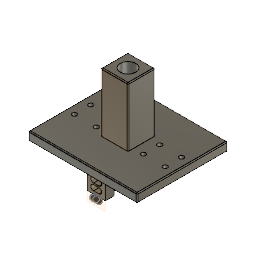
camera_house (Autodesk Fusion 360 design; units mm, degrees)
Autodesk Fusion 360 part; units mm, degrees
sketch "Sketch1" plane through (0, 0, 0) normal (0, 0, 1) x (1, 0, 0)
  line L0 (0, 0) -> (120, 0)
  line L1 (120, 0) -> (120, 100)
  line L2 (120, 100) -> (0, 100)
  line L3 (0, 100) -> (0, 0)
  line L4 (60, 100) -> (60, 0)
  line L5 (98, 100) -> (98, 0)
  line L6 (22, 100) -> (22, 0)
  line L7 (22, 50) -> (10, 50)
  line L8 (10, 50) -> (10, 59)
  line L9 (10, 59) -> (22, 59)
  line L10 (22, 59) -> (22, 50)
  circle A0 centre (10, 59) radius 2.5
  line L11 (22, 50) -> (34, 50)
  line L12 (34, 50) -> (34, 59)
  line L13 (34, 59) -> (22, 59)
  line L14 (22, 59) -> (22, 50)
  line L15 (10, 50) -> (34, 50)
  line L16 (34, 50) -> (34, 41)
  line L17 (34, 41) -> (10, 41)
  line L18 (10, 41) -> (10, 50)
  circle A1 centre (10, 41) radius 2.5
  circle A2 centre (34, 41) radius 2.5
  circle A3 centre (34, 59) radius 2.5
  line L19 (60, 50) -> (120, 50)
  line L20 (98, 50) -> (110, 50)
  line L21 (110, 50) -> (110, 59)
  line L22 (110, 59) -> (98, 59)
  line L23 (98, 59) -> (98, 50)
  line L24 (98, 50) -> (86, 50)
  line L25 (86, 50) -> (86, 59)
  line L26 (86, 59) -> (98, 59)
  line L27 (98, 59) -> (98, 50)
  line L28 (86, 50) -> (110, 50)
  line L29 (110, 50) -> (110, 41)
  line L30 (110, 41) -> (86, 41)
  line L31 (86, 41) -> (86, 50)
  circle A4 centre (86, 59) radius 2.5
  circle A5 centre (110, 59) radius 2.5
  circle A6 centre (86, 41) radius 2.5
  circle A7 centre (110, 41) radius 2.5
  dimension "d1" = 120
  dimension "d2" = 100
  dimension "d3" = 38
  dimension "d4" = 38
  dimension "d6" = 5
  dimension "d7" = 24
  dimension "d8" = 18
  dimension "d9" = 5
  dimension "d10" = 5
  dimension "d11" = 5
  dimension "d12" = 9
  dimension "d13" = 12
  dimension "d14" = 9
  dimension "d15" = 12
  dimension "d16" = 24
  dimension "d17" = 9
  dimension "d18" = 5
  dimension "d19" = 5
  dimension "d20" = 5
  dimension "d21" = 5
  constraint horizontal L0
  constraint vertical L1
  constraint horizontal L2
  constraint vertical L3
  constraint coincident L0.start L3.end
  constraint midpoint L2 L4.start
  constraint midpoint L0 L4.end
  constraint coincident L2 L5.start
  constraint coincident L0 L5.end
  constraint perpendicular L0 L5
  constraint coincident L2 L6.start
  constraint coincident L0 L6.end
  constraint perpendicular L0 L6
  constraint horizontal L7
  constraint vertical L8
  constraint horizontal L9
  constraint vertical L10
  constraint midpoint L6 L7.start
  constraint coincident L8.end L9.start
  constraint horizontal L11
  constraint vertical L12
  constraint horizontal L13
  constraint vertical L14
  constraint horizontal L15
  constraint vertical L16
  constraint horizontal L17
  constraint vertical L18
  constraint coincident L17.end L18.start
  constraint coincident L16.end L17.start
  constraint coincident L12.end L13.start
  constraint midpoint L4 L19.start
  constraint midpoint L1 L19.end
  constraint horizontal L20
  constraint vertical L21
  constraint horizontal L22
  constraint vertical L23
  constraint midpoint L5 L20.start
  constraint horizontal L24
  constraint vertical L25
  constraint horizontal L26
  constraint vertical L27
  constraint horizontal L28
  constraint vertical L29
  constraint horizontal L30
  constraint vertical L31
  constraint coincident L25.end L26.start
  constraint coincident L21.end L22.start
  constraint coincident L30.end L31.start
  constraint coincident L29.end L30.start
  measures "d1" distance of L0.start L0.end
  measures "d2" distance of L0.start L2.end
  measures "d3" distance of L4 L5
  measures "d4" distance of L4 L6
  measures "d6" diameter of A0
  measures "d7" distance of L8 L12
  measures "d8" distance of L9 L17
  measures "d9" diameter of A1
  measures "d10" diameter of A2
  measures "d11" diameter of A3
  measures "d12" distance of L20.start L22.end
  measures "d13" distance of L20.start L20.end
  measures "d14" distance of L20.start L22.end
  measures "d15" distance of L20.start L24.end
  measures "d16" distance of L24.end L20.end
  measures "d17" distance of L24.end L30.end
  measures "d18" diameter of A4
  measures "d19" diameter of A5
  measures "d20" diameter of A6
  measures "d21" diameter of A7
  measures "d40" diameter of L0.end
extrude "Extrude1" add sketch "Sketch1" along normal blind 10 contours L0 L2 L3 L6 L8 L9 A0 L17 L18 A1 | L0 L2 L4 L6 L12 L13 L16 L17 A2 A3 | L0 L4 L5 L19 L30 L31 A6 | L6 L7 L15 L17 L18 A1 | L6 L11 L15 L16 L17 A2 | L0 L1 L5 L19 L29 L30 A7 | L2 L4 L5 L19 L25 L26 A4 | L6 L7 L8 L9 L10 A0 L14 L15 | L6 L10 L11 L12 L13 L14 L15 A3 | L5 L19 L24 L28 L30 L31 A6 | L5 L19 L20 L28 L29 L30 A7 | L5 L19 L23 L24 L25 L26 L27 L28 A4 | L1 L2 L5 L19 L21 L22 A5 | L5 L19 L20 L21 L22 L23 L27 L28 A5
sketch "Sketch2" plane through (0, 0, 0) normal (0, 0, -1) x (1, 0, 0)
  circle A0 centre (110, -41) radius 2.5
  circle A1 centre (86, -59) radius 2.5
  circle A2 centre (10, -59) radius 2.5
  circle A3 centre (110, -59) radius 2.5
  circle A4 centre (86, -41) radius 2.5
  circle A5 centre (10, -41) radius 2.5
  circle A6 centre (34, -41) radius 2.5
  circle A7 centre (34, -59) radius 2.5
  line L0 (0, 0) -> (0, -100)
  line L1 (0, -100) -> (120, -100)
  line L2 (120, -100) -> (120, 0)
  line L3 (120, 0) -> (0, 0)
  line L4 (0, -50) -> (120, -50)
  line L5 (60, -100) -> (60, 0)
  line L6 (0, -85) -> (120, -85)
  line L7 (60, -85) -> (70, -85)
  line L8 (70, -85) -> (70, -75)
  line L9 (70, -75) -> (60, -75)
  line L10 (60, -75) -> (60, -85)
  line L11 (60, -85) -> (50, -85)
  line L12 (50, -85) -> (50, -75)
  line L13 (50, -75) -> (60, -75)
  line L14 (60, -75) -> (60, -85)
  line L15 (0, -15) -> (120, -15)
  line L16 (60, -15) -> (70, -15)
  line L17 (70, -15) -> (70, -25)
  line L18 (70, -25) -> (60, -25)
  line L19 (60, -25) -> (60, -15)
  line L20 (60, -25) -> (50, -25)
  line L21 (50, -25) -> (50, -15)
  line L22 (50, -15) -> (60, -15)
  line L23 (60, -15) -> (60, -25)
  dimension "d24" = 15
  dimension "d25" = 10
  dimension "d26" = 10
  dimension "d27" = 10
  dimension "d28" = 15
  dimension "d29" = 10
  dimension "d30" = 10
  dimension "d31" = 10
  dimension "d32" = 10
  constraint midpoint L0 L4.start
  constraint midpoint L2 L4.end
  constraint midpoint L1 L5.start
  constraint midpoint L3 L5.end
  constraint coincident L0 L6.start
  constraint coincident L2 L6.end
  constraint horizontal L7
  constraint vertical L8
  constraint horizontal L9
  constraint vertical L10
  constraint midpoint L6 L7.start
  constraint horizontal L11
  constraint vertical L12
  constraint horizontal L13
  constraint vertical L14
  constraint coincident L0 L15.start
  constraint coincident L2 L15.end
  constraint horizontal L16
  constraint vertical L17
  constraint horizontal L18
  constraint vertical L19
  constraint midpoint L15 L16.start
  constraint horizontal L20
  constraint vertical L21
  constraint horizontal L22
  constraint vertical L23
  measures "d24" distance of L1 L6
  measures "d25" distance of L7.start L7.end
  measures "d26" distance of L7.start L9.end
  measures "d27" distance of L7.start L9.end
  measures "d28" distance of L3 L15
  measures "d29" distance of L16.start L16.end
  measures "d30" distance of L16.start L18.end
  measures "d31" distance of L18.end L20.end
  measures "d32" distance of L18.end L16.start
extrude "Extrude2" add sketch "Sketch2" along normal blind 20 contours L5 L15 L19 L20 L21 L22 L23 | L5 L15 L16 L17 L18 L19 L23 | L5 L6 L10 L11 L12 L13 L14 | L5 L6 L7 L8 L9 L10 L14
extrude "Extrude3" add 2 faces at (56.6667, 18.3333, -20) (56.6667, 78.3333, -20) along direction (0, 0, -1) blind 10
sketch "Sketch6" plane through (0, 15, 0) normal (0, -1, 0) x (1, 0, 0)
  line L0 (70, 0) -> (50, 0)
  line L1 (50, 0) -> (50, -30)
  line L2 (50, -30) -> (70, -30)
  line L3 (70, -30) -> (70, 0)
  line L4 (50, -15.9999) -> (70, -16)
  line L5 (56.995, -26.5146) -> (62.9949, -26.5247)
  arc A0 (62.9949, -26.5247) -> (63.0051, -20.5247) centre (63, -23.5247) ccw
  line L6 (63.0051, -20.5247) -> (57.0051, -20.5146)
  arc A1 (57.0051, -20.5146) -> (56.995, -26.5146) centre (57, -23.5146) ccw
  line L7 (50, -23.5028) -> (54, -23.5096)
  line L8 (66, -23.5298) -> (70, -23.5365)
  line L9 (57, -11.4803) -> (63, -11.4803)
  arc A2 (63, -11.4803) -> (63, -5.4803) centre (63, -8.4803) ccw
  line L10 (63, -5.4803) -> (57, -5.4803)
  arc A3 (57, -5.4803) -> (57, -11.4803) centre (57, -8.4803) ccw
  line L11 (50, -8.4803) -> (54, -8.4803)
  line L12 (66, -8.4803) -> (70, -8.4803)
  point P0 (60, -23.5197)
  point P1 (60, -8.4803)
  dimension "d40" = 6
  dimension "d41" = 6
  constraint coincident L1 L4.start
  constraint coincident L3 L4.end
  constraint coincident L1 L11.start
  constraint coincident L3 L12.end
  constraint perpendicular L3 L11
  constraint coincident L1 L7.start
  constraint coincident L3 L8.end
  constraint tangent L5 A0
  constraint tangent A0 L6
  constraint parallel L5 L6
  constraint tangent L6 A1
  constraint tangent L5 A1
  constraint coincident A1 L7.end
  constraint coincident A0 L8.start
  constraint collinear L7 L8
  constraint coincident P0 L7
  constraint tangent L9 A2
  constraint tangent A2 L10
  constraint parallel L9 L10
  constraint tangent L10 A3
  constraint tangent L9 A3
  constraint coincident A3 L11.end
  constraint coincident A2 L12.start
  constraint collinear L11 L12
  constraint coincident P1 L11
  measures "d40" diameter of A0
  measures "d41" diameter of A2
extrude "Extrude4" cut sketch "Sketch6" against normal blind 200 contours L9 A2 L10 A3 | L5 A0 L6 A1
extrude "Extrude5" add 2 faces at (56.6667, 78.3333, -30) (56.6667, 18.3333, -30) along direction (0, 0, -1) blind 10
sketch "Sketch7" plane through (0, 15, 0) normal (0, -1, 0) x (1, 0, 0)
  line L0 (63, -11.4803) -> (57, -11.4803)
  arc A0 (57, -5.4803) -> (57, -11.4803) centre (57, -8.4803) ccw
  line L1 (57, -5.4803) -> (63, -5.4803)
  arc A1 (63, -11.4803) -> (63, -5.4803) centre (63, -8.4803) ccw
  line L2 (62.9949, -26.5247) -> (56.995, -26.5146)
  arc A2 (57.0051, -20.5146) -> (56.995, -26.5146) centre (57, -23.5146) ccw
  line L3 (57.0051, -20.5146) -> (63.0051, -20.5247)
  arc A3 (62.9949, -26.5247) -> (63.0051, -20.5247) centre (63, -23.5247) ccw
  line L4 (70, 0) -> (50, 0)
  line L5 (50, 0) -> (50, -40)
  line L6 (50, -40) -> (70, -40)
  line L7 (70, -40) -> (70, 0)
  line L8 (57, -36) -> (63, -36)
  arc A4 (63, -36) -> (63, -30) centre (63, -33) ccw
  line L9 (63, -30) -> (57, -30)
  arc A5 (57, -30) -> (57, -36) centre (57, -33) ccw
  line L10 (57, -33) -> (63, -33) construction
  point P0 (60, -33)
  dimension "d46" = 6
  constraint tangent L8 A4
  constraint tangent A4 L9
  constraint parallel L8 L9
  constraint tangent L9 A5
  constraint tangent L8 A5
  constraint horizontal L10
  constraint midpoint L10 P0
  measures "d46" diameter of A4
sketch "Sketch8" plane through (0, 0, 10) normal (0, 0, 1) x (-1, 0, 0)
  circle A0 centre (-110, -41) radius 2.5
  circle A1 centre (-86, -59) radius 2.5
  circle A2 centre (-10, -59) radius 2.5
  circle A3 centre (-110, -59) radius 2.5
  circle A4 centre (-86, -41) radius 2.5
  circle A5 centre (-10, -41) radius 2.5
  circle A6 centre (-34, -41) radius 2.5
  circle A7 centre (-34, -59) radius 2.5
  line L0 (0, -100) -> (0, 0)
  line L1 (0, 0) -> (-120, 0)
  line L2 (-120, 0) -> (-120, -100)
  line L3 (-120, -100) -> (0, -100)
  line L4 (-60, 0) -> (-60, -100)
  line L5 (0, -50) -> (-120, -50)
  line L6 (-86, -59) -> (-86, -100)
  line L7 (-80.75, -100) -> (-80.75, -11.2422)
  line L8 (-60, -50) -> (-75, -50)
  line L9 (-75, -50) -> (-75, -65)
  line L10 (-75, -65) -> (-60, -65)
  line L11 (-60, -65) -> (-60, -50)
  line L12 (-60, -50) -> (-45, -50)
  line L13 (-45, -50) -> (-45, -65)
  line L14 (-45, -65) -> (-60, -65)
  line L15 (-60, -65) -> (-60, -50)
  line L16 (-45, -50) -> (-75, -50)
  line L17 (-75, -50) -> (-75, -35)
  line L18 (-75, -35) -> (-45, -35)
  line L19 (-45, -35) -> (-45, -50)
  dimension "d51" = 26
  dimension "d52" = 5.25
  dimension "d53" = 30
  dimension "d54" = 15
  constraint midpoint L1 L4.start
  constraint midpoint L3 L4.end
  constraint midpoint L0 L5.start
  constraint midpoint L2 L5.end
  constraint coincident A1.centre L6.start
  constraint coincident L3 L6.end
  constraint perpendicular L3 L6
  constraint coincident L3 L7.start
  constraint perpendicular L3 L7
  constraint horizontal L8
  constraint vertical L9
  constraint horizontal L10
  constraint vertical L11
  constraint midpoint L4 L8.start
  constraint horizontal L12
  constraint vertical L13
  constraint horizontal L14
  constraint vertical L15
  constraint horizontal L16
  constraint vertical L17
  constraint horizontal L18
  constraint vertical L19
  measures "d51" distance of A4.centre L4
  measures "d52" distance of L6 L7
  measures "d53" distance of L12.end L8.end
  measures "d54" distance of L12.end L18.end
extrude "Extrude8" add sketch "Sketch8" along normal blind 65 contours L4 L5 L11 L12 L13 L14 L15 L16 | L4 L5 L12 L16 L18 L19 | L4 L5 L8 L9 L10 L11 L15 L16 | L4 L5 L8 L16 L17 L18
sketch "Sketch9" plane through (0, 0, 75) normal (0, 0, 1) x (-1, 0, 0)
  line L0 (-75, -35) -> (-75, -65)
  line L1 (-75, -65) -> (-45, -65)
  line L2 (-45, -65) -> (-45, -35)
  line L3 (-45, -35) -> (-75, -35)
  line L4 (-60, -35) -> (-60, -65)
  line L5 (-45, -50) -> (-75, -50)
  circle A0 centre (-60, -50) radius 8.5
  dimension "d57" = 17
  constraint midpoint L3 L4.start
  constraint midpoint L1 L4.end
  constraint midpoint L2 L5.start
  constraint midpoint L0 L5.end
  constraint midpoint L5 A0.centre
  measures "d57" diameter of A0
extrude "Extrude9" cut sketch "Sketch9" against normal blind 80 contours L4 L5 A0 | L4 L5 A0 | L4 L5 A0 | L4 L5 A0
sketch "Sketch10" plane through (0, 15, 0) normal (0, -1, 0) x (1, 0, 0)
  line L0 (50, -29.8136) -> (70, -29.8136)
  line L1 (70, -29.8136) -> (70, -40)
  line L2 (70, -40) -> (50, -40)
  line L3 (50, -40) -> (50, -29.8136)
  line L4 (50, 0) -> (50, -40)
  line L5 (63, -5.4803) -> (57, -5.4803)
  line L6 (56.995, -26.5146) -> (62.9949, -26.5247)
  line L7 (60, -5.4803) -> (59.9949, -26.5197)
  line L8 (70, 0) -> (70, -40)
  line L9 (70, -16) -> (50, -16)
  line L10 (56.9968, -18.9993) -> (62.9968, -19.0007)
  arc A0 (62.9968, -19.0007) -> (62.9982, -13.0007) centre (62.9975, -16.0007) ccw
  line L11 (62.9982, -13.0007) -> (56.9982, -12.9993)
  arc A1 (56.9982, -12.9993) -> (56.9968, -18.9993) centre (56.9975, -15.9993) ccw
  line L12 (56.9975, -15.9993) -> (62.9975, -16.0007) construction
  point P0 (70, -40)
  point P1 (59.9975, -16)
  dimension "d60" = 6
  constraint horizontal L0
  constraint vertical L1
  constraint horizontal L2
  constraint vertical L3
  constraint coincident P0 L1.end
  constraint coincident L0.start L4
  constraint midpoint L5 L7.start
  constraint midpoint L6 L7.end
  constraint coincident L8 L9.start
  constraint coincident L4 L9.end
  constraint perpendicular L4 L9
  constraint tangent L10 A0
  constraint tangent A0 L11
  constraint parallel L10 L11
  constraint tangent L11 A1
  constraint tangent L10 A1
  constraint perpendicular L7 L12
  constraint midpoint L7 P1
  constraint midpoint L12 P1
  measures "d60" diameter of A0
extrude "Extrude10" cut sketch "Sketch10" against normal blind 200 contours L0 L1 L2 L3 L4 L8 | L7 L9 L11 A1 | L7 L9 L10 A1 | L7 L9 L10 A0 | L7 L9 A0 L11
sketch "Sketch11" plane through (0, 35, 0) normal (0, -1, 0) x (1, 0, 0)
  line L0 (45, 10) -> (75, 10)
  line L1 (75, 10) -> (75, 75)
  line L2 (75, 75) -> (45, 75)
  line L3 (45, 75) -> (45, 10)
fillet "Fillet1" radius 1 20 edges at (75, 50, 75) (60, 65, 75) (60, 35, 75) (45, 50, 75) (75, 35, 42.5) (75, 65, 42.5) (45, 65, 42.5) (45, 35, 42.5) (0, 50, 10) (60, 100, 10) (0, 100, 5) (0, 50, 0) (60, 100, 0) (60, 0, 10) (60, 0, 0) (0, 0, 5) (120, 0, 5) (120, 50, 10) (120, 50, 0) (120, 100, 5)
extrude "Extrude6" [suppressed]
sketch "Sketch5" plane through (0, 15, 0) normal (0, -1, 0) x (1, 0, 0)
sketch "Sketch4" plane through (0, 15, 0) normal (0, -1, 0) x (1, 0, 0)
  line L0 (70, 0) -> (50, 0)
  line L1 (50, 0) -> (50, -30)
  line L2 (50, -30) -> (70, -30)
  line L3 (70, -30) -> (70, 0)
  line L4 (50, 0) -> (50, -20)
  line L5 (50, -10) -> (70, -10)
  line L6 (50, -21.4872) -> (70, -21.4747)
  line L7 (50, -16) -> (70, -16)
  dimension "d39" = 6
  constraint midpoint L4 L5.start
  constraint coincident L3 L5.end
  constraint coincident L1 L6.start
  constraint coincident L3 L6.end
  measures "d39" distance of L5 L7
